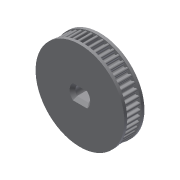
# Autodesk Inventor part: 00_Pulley_28byj-48
Saved by Autodesk Inventor 2019.4 (Build 234330000, 330)
## iProperties
Created: 2021-10-06
Part Number: 00_Pulley_28byj-48
Material: Generic
Document SubType Name: Modeling
Designer: diederichbenedict
Density: 1 g/cm^3
Appearance: Default
Author: diederichbenedict
Autodesk Inventor part; units mm, degrees
ref_plane "YZ Plane" through (0, 0, 0) normal (1, 0, 0) x (0, 1, 0)
ref_plane "XZ Plane" through (0, 0, 0) normal (0, 1, 0) x (-1, 0, 0)
ref_plane "XY Plane" through (0, 0, 0) normal (0, 0, 1) x (1, 0, 0)
sketch "Sketch1" plane through (0, 0, 0) normal (0, 0, 1) x (1, 0, 0)
  arc A0 (-2, 3) -> (-2, 0) centre (0, 1.5) ccw projected
  arc A1 (2, 0) -> (2, 3) centre (0, 1.5) ccw projected
  line L0 (-2, 0) -> (2, 0) projected
  line L1 (2, 3) -> (-2, 3) projected
  arc A2 (2.0494, -0.1) -> (2.0494, 3.1) centre (0, 1.5) ccw
  line L2 (2.0494, -0.1) -> (-2.0494, -0.1)
  arc A3 (-2.0494, 3.1) -> (-2.0494, -0.1) centre (0, 1.5) ccw
  line L3 (-2.0494, 3.1) -> (2.0494, 3.1)
  circle A4 centre (0, 1.5) radius 14
  point P0 (0, 0)
  dimension "d0" = 0.1
  dimension "d1" = 28
  constraints: 4 end point, 4 point on circle, 3 centre point, 1 coincident, 3 other
  measures "d0" radial gap between concentric circles of A1 A2
  measures "d1" diameter of A4
extrude "Extrusion1" add sketch "Sketch1" along normal blind 8 contours A4
sketch "Sketch2" plane through (0, 1.5, 8) normal (0, 0, 1) x (1, 0, 0)
  circle A0 centre (0, 0) radius 14 projected
  line L0 (0.45, -15.25) -> (-0.45, -15.25)
  line L1 (-0.45, -15.25) -> (-0.45, -12.75)
  line L2 (-0.45, -12.75) -> (0.45, -12.75)
  line L3 (0.45, -12.75) -> (0.45, -15.25)
  circle A1 centre (0, 0) radius 14 projected
  line L4 (0.45, -15.25) -> (-0.45, -12.75) construction
  line L5 (-0.45, -15.25) -> (0.45, -12.75) construction
  point P0 (0, -1.5)
  point P1 (0, -14)
  dimension "d4" = 0.9
  dimension "d5" = 2.5
  constraints: 12 end point, 2 midpoint, 2 parallel, 1 horizontal, 1 perpendicular, 1 vertical alignment, 1 other
  measures "d4" distance of L1.end L2.end
  measures "d5" distance of L0.end L1.end
extrude "Extrusion2" add sketch "Sketch2" against normal up to surface (8 mm away) contours L1 L2 L3 A0 | A0 L3 L0 L1 picked at (-0.05, -13.1664)
fillet "Fillet1" radius 0.4 4 edges at (-0.45, -13.75, 4) (0.45, -13.75, 4) (-0.45, -12.4928, 4) (0.45, -12.4928, 4)
pattern_circular "Circular Pattern1" count 48 over 360 about axis through (0, 1.5, 0) along (0, 0, 1) of "Extrusion2", "Fillet1"
sketch "Sketch3" plane through (0, 0, 8) normal (0, 0, 1) x (1, 0, 0)
  arc A0 (2.0494, -0.1) -> (2.0494, 3.1) centre (0, 1.5) ccw projected
  circle A1 centre (0, 1.5) radius 15.5
  line L0 (2.0494, -0.1) -> (-2.0494, -0.1) projected
  arc A2 (-2.0494, 3.1) -> (-2.0494, -0.1) centre (0, 1.5) ccw projected
  line L1 (-2.0494, 3.1) -> (2.0494, 3.1) projected
  point P0 (0, 0)
  dimension "d20" = 31
  constraints: 1 centre point, 1 coincident
  measures "d20" diameter of A1
extrude "Extrusion3" add sketch "Sketch3" against normal blind 1
pattern_linear "Rectangular Pattern1" count 2 spacing 8 along (0, 0, -1) of "Extrusion3"
chamfer "Chamfer1" distance 1 angle 45 4 edges at (-2.6, 1.5, 8) (0, -0.1, 8) (2.6, 1.5, 8) (0, 3.1, 8)
body "Solid1"
